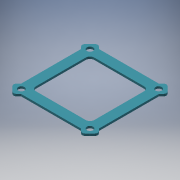
# Autodesk Inventor part: Base
Saved by Autodesk Inventor 2016 (Build 200138000, 138)
## iProperties
Created: 2015-03-29
Part Number: Base
Material: PC/ABS Plastic
Document SubType Name: Modeling
Designer: Erin
Density: 0.357273 g/cm^3
Appearance: Cadet Blue
Mass: 3.14413 g
Surface Area: 66.4965 cm^2
Volume: 5.71659 cm^3
Author: Erin
Autodesk Inventor part; units mm, degrees
ref_plane "YZ Plane" through (0, 0, 0) normal (1, 0, 0) x (0, 1, 0)
ref_plane "XZ Plane" through (0, 0, 0) normal (0, 1, 0) x (-1, 0, 0)
ref_plane "XY Plane" through (0, 0, 0) normal (0, 0, 1) x (1, 0, 0)
sketch "Sketch1" plane through (0, 0, 0) normal (0, 0, 1) x (1, 0, 0)
  line L0 (-48, 48) -> (48, 48)
  line L1 (48, 48) -> (48, -48)
  line L2 (48, -48) -> (-48, -48)
  line L3 (-48, -48) -> (-48, 48)
  line L4 (38, 38) -> (-38, 38)
  line L5 (-38, 38) -> (-38, -38)
  line L6 (-38, -38) -> (38, -38)
  line L7 (38, -38) -> (38, 38)
  line L8 (0, 152.7233) -> (0, -72.1628) construction
  line L9 (-77.8847, 0) -> (88.8171, 0) construction
  line L10 (-48, 43) -> (48, 43) construction
  line L11 (-43, 48) -> (-43, -48) construction
  line L12 (-48, -43) -> (48, -43) construction
  circle A0 centre (-43, 25) radius 2.25
  circle A1 centre (-43, -25) radius 2.25
  circle A2 centre (-43, -43) radius 2.25
  circle A3 centre (-43, 43) radius 2.25
  line L13 (-48, 30) -> (48, 30) construction
  line L14 (-48, -30) -> (48, -30) construction
  line L15 (-50, 31) -> (-36, 31)
  line L16 (-36, 31) -> (-36, -31)
  line L17 (-36, -31) -> (-50, -31)
  line L18 (-50, -31) -> (-50, 31)
  point P0 (0, 0)
  point P1 (0, 48)
  point P2 (48, 0)
  dimension "d0" = 96
  dimension "d1" = 96
  dimension "d2" = 10
  dimension "d5" = 5
  dimension "d11" = 5
  dimension "d14" = 5
  dimension "d31" = 4.5
  dimension "d32" = 4.5
  dimension "d61" = 4.5
  dimension "d62" = 4.5
  dimension "d65" = 30
  dimension "d66" = 30
  dimension "d67" = 5
  dimension "d68" = 5
  dimension "d74" = 1
  dimension "d75" = 1
  dimension "d76" = 2
  dimension "d77" = 2
  constraints: 38 end point, 16 point on line, 9 perpendicular, 7 parallel, 4 centre point, 3 horizontal, 2 midpoint, 1 horizontal alignment, 1 vertical, 1 vertical alignment, 3 other
  measures "d0" distance of L1.end L2.end
  measures "d1" distance of L0.end L1.end
  measures "d2" distance between parallel lines of L4 L0
  measures "d5" distance between parallel lines of L10 L0
  measures "d11" distance between parallel lines of L11 L3
  measures "d14" distance between parallel lines of L12 L2
  measures "d31" diameter of A0
  measures "d32" diameter of A1
  measures "d61" diameter of A2
  measures "d62" diameter of A3
  measures "d65" distance between parallel lines of L13 L9
  measures "d66" distance between parallel lines of L14 L9
  measures "d67" distance from line of A1.centre L14
  measures "d68" distance from line of A0.centre L13
  measures "d74" distance between parallel lines of L13 L15
  measures "d75" distance between parallel lines of L17 L14
  measures "d76" distance between parallel lines of L3 L18
  measures "d77" distance between parallel lines of L16 L5
sketch "Sketch3" plane through (0, 0, 0) normal (0, 0, 1) x (1, 0, 0)
  circle A0 centre (-43, 43) radius 2.25 projected
  circle A1 centre (-43, -43) radius 2.25 projected
  line L0 (48, -48) -> (-48, -48) projected
  line L1 (-48, -48) -> (-48, 48) projected
  line L2 (-38, -38) -> (38, -38) projected
  line L3 (-38, 38) -> (-38, -38) projected
  line L4 (38, 38) -> (-38, 38) projected
  line L5 (-48, 48) -> (48, 48) projected
  line L6 (0, 62.8599) -> (0, -69.2948) construction
  line L7 (-75.2692, 0) -> (82.2152, 0) construction
  line L8 (-28, 28) -> (28, 28)
  line L9 (28, 28) -> (28, -28)
  line L10 (28, -28) -> (-28, -28)
  line L11 (-28, -28) -> (-28, 28)
  line L12 (38, -38) -> (38, 38) projected
  line L13 (48, 48) -> (48, -48) projected
  line L14 (-31.0678, -24.7038) -> (24.7038, 31.0678)
  line L15 (24.7038, 31.0678) -> (31.0678, 24.7038)
  line L16 (31.0678, 24.7038) -> (-24.7038, -31.0678)
  line L17 (-24.7038, -31.0678) -> (-31.0678, -24.7038)
  line L18 (-37.8254, -37.8254) -> (27.8858, 27.8858) construction
  line L19 (-3.182, 3.182) -> (3.182, -3.182) construction
  line L20 (-48, -48) -> (-29.3, -48)
  line L21 (-29.3, -48) -> (-29.3, -29.3)
  line L22 (-29.3, -29.3) -> (-48, -29.3)
  line L23 (-48, -29.3) -> (-48, -48)
  line L24 (-35.664, -29.3) -> (-25.0574, -18.6934)
  line L25 (-25.0574, -18.6934) -> (-18.6934, -25.0574)
  line L26 (-18.6934, -25.0574) -> (-29.3, -35.664)
  line L27 (-29.3, -35.664) -> (-35.664, -29.3)
  line L28 (-32.482, -32.482) -> (-21.8754, -21.8754) construction
  line L29 (-30.3607, -23.9967) -> (-23.9967, -30.3607) construction
  circle A2 centre (-24.7038, -24.7038) radius 2.25
  line L30 (-21, 21) -> (21, 21)
  line L31 (21, 21) -> (21, -21)
  line L32 (21, -21) -> (-21, -21)
  line L33 (-21, -21) -> (-21, 21)
  point P0 (0, 0)
  point P1 (0, 0)
  point P2 (0, 21)
  point P3 (0, 28)
  point P4 (21, 0)
  point P5 (28, 0)
  dimension "d80" = 9
  dimension "d81" = 18.7
  dimension "d83" = 10
  dimension "d84" = 10
  dimension "d85" = 10
  dimension "d86" = 10
  dimension "d98" = 15
  dimension "d99" = 9
  dimension "d100" = 4.5
  dimension "d101" = 4
  dimension "d102" = 1
  dimension "d108" = 18.7
  dimension "d113" = 42
  dimension "d114" = 42
  constraints: 52 end point, 12 midpoint, 10 parallel, 5 horizontal, 5 perpendicular, 5 point on line, 2 vertical, 1 centre point, 1 coincident, 1 horizontal alignment, 1 vertical alignment
  measures "d80" distance of L14.end L15.end
  measures "d81" distance of L21.end L22.end
  measures "d83" distance between parallel lines of L3 L11
  measures "d84" distance between parallel lines of L4 L8
  measures "d85" distance between parallel lines of L12 L9
  measures "d86" distance between parallel lines of L2 L10
  measures "d98" distance of L25.end L26.end
  measures "d99" distance of L24.end L25.end
  measures "d100" diameter of A2
  measures "d101" distance from line of A2.centre L25
  measures "d102" distance between parallel lines of L29 L17
  measures "d108" distance of L20.end L21.end
  measures "d113" distance of L30.start L30.end
  measures "d114" distance of L30.end L31.end
extrude "Extrusion7" add sketch "Sketch3" along normal blind 1.5 contours L16 L32 L31 L9 L10 | L10 L17 L11 L14 L25 L16 | L10 L11 L17 | L25 L14 L33 L32 L16 | L11 L8 L14 L30 L33 | L16 L31 L30 L14 L8 L15 L9 | L32 L33 L14 L30 L31 L16 | L16 L31 L32 | L15 L8 L9 | L33 L30 L14 | A2
extrude "Extrusion9" add sketch "Sketch3" along normal blind 1.5 contours L17 L10 L16 | L10 L17 L11 L14 L25 L16 | L14 L11 L17 | L25 L14 L33 L32 L16 | L16 L31 L30 L14 L8 L15 L9 | L9 L15 L16 | L32 L33 L14 L30 L31 L16 | L14 L15 L8 | A2
mirror "Mirror6" about plane through (0, 0, 0) normal (1, 0, 0) of "Extrusion9"
extrude "Extrusion10" cut sketch "Sketch3" along normal blind 10 contours A2
pattern_circular "Circular Pattern3" count 4 over 360 about axis through (0, 0, -10) along (0, 0, 1) of "Extrusion10"
fillet "Fillet2" radius 2 2 edges at (-24.7038, -31.0678, 0.75) (-31.0678, -24.7038, 0.75)
pattern_circular "Circular Pattern4" count 4 over 360 about axis through (0, 0, -10) along (0, 0, 1) of "Fillet2"
extrude "Extrusion11" cut sketch "Sketch3" along normal blind 10 contours L32 L33 L14 L30 L31 L16 | L16 L31 L32 | L33 L30 L14
fillet "Fillet3" radius 3 4 edges at (-21, 21, 0.75) (21, 21, 0.75) (21, -21, 0.75) (-21, -21, 0.75)
equation "\"d31\" = screw"
equation "\"d32\" = screw"
equation "\"d61\" = screw"
equation "\"d62\" = screw"
equation "\"screw\" = 4.5"
body "Solid2"
